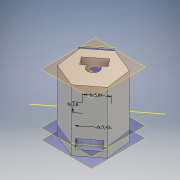
# Autodesk Inventor part: wheel_to_motor
Saved by Autodesk Inventor 2017 (Build 210142000, 142)
## iProperties
Created: 2017-09-26
Part Number: wheel_to_motor
Material: Generic
Document SubType Name: Modeling
Designer: fabre
Density: 1 g/cm^3
Appearance: Default
Author: fabre
Autodesk Inventor part; units mm, degrees
ref_plane "YZ Plane" through (0, 0, 0) normal (1, 0, 0) x (0, 1, 0)
ref_plane "XZ Plane" through (0, 0, 0) normal (0, 1, 0) x (-1, 0, 0)
ref_plane "XY Plane" through (0, 0, 0) normal (0, 0, 1) x (1, 0, 0)
sketch "Sketch2" plane through (0, 0, 0) normal (0, 0, 1) x (1, 0, 0)
  circle A0 centre (0, 0) radius 7.1 construction
  line L0 (-0.9625, 7.0345) -> (5.6108, 4.3508)
  line L1 (5.6108, 4.3508) -> (6.5733, -2.6837)
  line L2 (6.5733, -2.6837) -> (0.9625, -7.0345)
  line L3 (0.9625, -7.0345) -> (-5.6108, -4.3508)
  line L4 (-5.6108, -4.3508) -> (-6.5733, 2.6837)
  line L5 (-6.5733, 2.6837) -> (-0.9625, 7.0345)
  dimension "wheel_hexa_d" = 14.2
  constraints: 12 end point, 6 point on circle, 5 equal length, 1 centre point, 1 coincident
  measures "wheel_hexa_d" diameter of A0
extrude "Extrusion1" add sketch "Sketch2" along normal blind 17
ref_plane "Work Plane1" through (0, 0, 2.89) normal (0, 0, -1) x (-1, 0, 0)
sketch "Sketch3" plane through (0, 0, 2.89) normal (0, 0, -1) x (-1, 0, 0)
  line L0 (6.5733, 2.6837) -> (0.9625, 7.0345) projected
  line L1 (-6.5733, -2.6837) -> (-0.9625, -7.0345) projected
  line L2 (0.9625, 7.0345) -> (6.5733, 2.6837) construction
  line L3 (3.7679, 4.8591) -> (-3.7679, -4.8591) construction
  line L4 (-0.9625, -7.0345) -> (-6.5733, -2.6837) construction
  circle A0 centre (0, 0) radius 3.715 construction
  line L5 (-3.4394, -1.4042) -> (-0.5036, -3.6807)
  line L6 (-0.5036, -3.6807) -> (2.9358, -2.2765)
  line L7 (2.9358, -2.2765) -> (3.4394, 1.4042)
  line L8 (3.4394, 1.4042) -> (0.5036, 3.6807)
  line L9 (0.5036, 3.6807) -> (-2.9358, 2.2765)
  line L10 (-2.9358, 2.2765) -> (-3.4394, -1.4042)
  dimension "d5" = 7.43
  constraints: 14 end point, 6 point on circle, 5 equal length, 2 midpoint, 1 centre point, 1 coincident, 1 parallel
  measures "d5" diameter of A0
ref_plane "Work Plane2" through (-6.5733, 2.6837, 17) normal (-0.6128, 0.7902, 0) x (0.7902, 0.6128, 0)
sketch "Sketch4" plane through (-6.5733, 2.6837, 17) normal (-0.6128, 0.7902, 0) x (0.7902, 0.6128, 0)
  line L0 (7.1, 17) -> (7.1, 0) construction
  line L1 (0, 17) -> (0, 0) construction
  line L2 (0, 17) -> (7.1, 17) construction
  line L3 (7.1, 0) -> (0, 0) construction
  line L4 (6.37, 15.41) -> (0.73, 15.41)
  line L5 (0.73, 15.41) -> (0.73, 12.81)
  line L6 (0.73, 12.81) -> (6.37, 12.81)
  line L7 (6.37, 12.81) -> (6.37, 15.41)
  line L8 (-9.8809, 14.11) -> (16.8778, 14.11) projected
  line L9 (7.1, 14.11) -> (0, 14.11) construction
  line L10 (3.55, 15.41) -> (3.55, 12.81) construction
  point P0 (3.55, 17)
  point P1 (-0.165, 14)
  point P2 (-0.165, 10)
  point P3 (3.55, 14.11)
  point P4 (6.37, 14.11)
  dimension "d13" = 5.64
  dimension "d14" = 2.6
  constraints: 12 end point, 5 midpoint, 5 point on line, 3 parallel, 1 horizontal, 1 perpendicular
  measures "d13" distance of L5.end L6.end
  measures "d14" distance of L4.end L5.end
extrude "Extrusion3" cut sketch "Sketch4" against normal up to surface (12.2976 mm away)
ref_plane "Work Plane3" through (0, 0, 0) normal (0, 0, -1) x (-1, 0, 0)
sketch "Sketch5" plane through (0, 0, 0) normal (0, 0, -1) x (-1, 0, 0)
  circle A0 centre (0, 0) radius 1.6
  dimension "vis_d" = 3.2
  constraints: 1 centre point, 1 coincident
  measures "vis_d" diameter of A0
extrude "Extrusion4" cut sketch "Sketch5" against normal blind 4.8
ref_plane "Work Plane4" through (0, 0, 17) normal (0, 0, 1) x (1, 0, 0)
sketch "Sketch6" plane through (0, 0, 17) normal (0, 0, 1) x (1, 0, 0)
  arc A0 (0.5392, 1.5064) -> (-1.5932, -0.1472) centre (0, 0) ccw construction
  line L0 (0.5392, 1.5064) -> (-1.5932, -0.1472)
  line L1 (-0.9625, 7.0345) -> (-6.5733, 2.6837) construction
  arc A1 (-1.5932, -0.1472) -> (0.5392, 1.5064) centre (0, 0) ccw
  line L2 (-2.7555, -1.0485) -> (-4.3487, 1.0062)
  line L3 (-4.3487, 1.0062) -> (0.1082, 4.4623)
  line L4 (0.1082, 4.4623) -> (1.7015, 2.4077)
  line L5 (1.7015, 2.4077) -> (-2.7555, -1.0485)
  line L6 (0, 0) -> (-3.7679, 4.8591) construction
  line L7 (-6.5733, 2.6837) -> (-0.9625, 7.0345) construction
  point P0 (-2.1202, 2.7343)
  dimension "d25" = 3.2
  dimension "d26" = 2.46
  dimension "petit_ecrou_cote" = 5.64
  dimension "petit_ecrou_depth" = 2.6
  dimension "d31" = 0
  constraints: 12 end point, 4 parallel, 4 point on circle, 2 centre point, 2 midpoint, 1 coincident, 1 perpendicular, 1 point on line
  measures "d25" diameter of A0
  measures "petit_ecrou_cote" distance of L4.end L2.start
  measures "petit_ecrou_depth" distance of L2.start L2.end
  measures "d31" distance between parallel lines of L0 L5
extrude "Extrusion5" cut sketch "Sketch6" against normal up to surface (12.81 mm away)
ref_plane "Work Plane5" through (-6.5733, 2.6837, 17) normal (-0.6128, 0.7902, 0) x (0.7902, 0.6128, 0)
sketch "Sketch7" plane through (-6.5733, 2.6837, 17) normal (-0.6128, 0.7902, 0) x (0.7902, 0.6128, 0)
  circle A0 centre (3.55, 3.82) radius 1.6
  line L0 (3.55, 3.82) -> (3.55, 0) construction
  line L1 (0.73, 0) -> (6.37, 0) construction
  point P0 (3.55, 17)
  dimension "d35" = 3.82
  dimension "d36" = 3.2
  constraints: 2 end point, 1 centre point, 1 midpoint, 1 vertical
  measures "d35" distance from line of L1 L0.start
  measures "d36" diameter of A0
extrude "Extrusion6" cut sketch "Sketch7" against normal up to surface (5.2888 mm away)
sketch "Sketch8" plane through (0, 0, 10) normal (0, 0, -1) x (-1, 0, 0)
  circle A0 centre (0, 0) radius 9.2875
  dimension "d40" = 18.575
  constraints: 1 centre point, 1 coincident
  measures "d40" diameter of A0
equation "\"big_hexa_depth\" = total_length"
equation "\"d5\" = ecrou_width"
equation "\"d13\" = petit_ecrou_cote"
equation "\"d14\" = petit_ecrou_depth"
equation "\"vis_d\" = vis_petit_ecrou_d"
equation "\"d25\" = vis_petit_ecrou_d"
equation "\"d32\" = petit_ecrou_hole_depth"
equation "\"d35\" = petit_ecrou_center_dist"
equation "\"d36\" = vis_petit_ecrou_d"
equation "\"d37\" = petit_ecrou_hole_depth"
equation "\"d40\" = 2.5 * ecrou_width"
equation "\"ecrou_dist\" = -vis_length_inside + 0.25 * petit_ecrou_hole_depth"
equation "\"ecrou_width\" = 7.43"
equation "\"ecrou_depth\" = 4"
equation "\"vis_petit_ecrou_d\" = 3.2"
equation "\"total_length\" = 17"
equation "\"d49\" = -vis_length_inside - petit_ecrou_cote"
equation "\"petit_ecrou_hole_depth\" = 7.64"
equation "\"petit_ecrou_center_dist\" = 3.82"
equation "\"vis_length_inside\" = 4.8"
body "Solid1"
